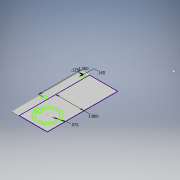
# Autodesk Inventor part: Power Button Plate
Saved by Autodesk Inventor 2019 (Build 230136000, 136)
## iProperties
Created: 2019-02-07
Part Number: Power Button Plate
Material: Generic
Document SubType Name: Modeling
Designer: mrhftc
Density: 1 g/cm^3
Appearance: Default
Author: mrhftc
Autodesk Inventor part; units mm, degrees
ref_plane "YZ Plane" through (0, 0, 0) normal (1, 0, 0) x (0, 1, 0)
ref_plane "XZ Plane" through (0, 0, 0) normal (0, 1, 0) x (-1, 0, 0)
ref_plane "XY Plane" through (0, 0, 0) normal (0, 0, 1) x (1, 0, 0)
sketch "Sketch1" plane through (0, 0, 0) normal (0, 1, 0) x (-1, 0, 0)
  line L0 (9.9313, 40.7784) -> (41.6813, 40.7784)
  line L1 (41.6813, 40.7784) -> (41.6813, 104.2784)
  line L2 (41.6813, 104.2784) -> (9.9313, 104.2784)
  line L3 (9.9313, 104.2784) -> (9.9313, 40.7784)
  point P0 (0, 0)
  dimension "d0" = 63.5
  dimension "d1" = 31.75
  constraints: 8 end point, 2 parallel, 1 horizontal, 1 perpendicular
  measures "d0" distance between parallel lines of L0 L2
  measures "d1" distance between parallel lines of L3 L1
extrude "Extrusion1" add sketch "Sketch1" along normal blind 0.3175
sketch "Sketch2" plane through (0, 0.3175, 0) normal (0, 1, 0) x (1, 0, 0)
  line L0 (-9.9313, -40.7784) -> (-41.6813, -40.7784) construction
  line L1 (-41.6813, -40.7784) -> (-41.6813, -104.2784) construction
  line L2 (-41.6813, -104.2784) -> (-9.9313, -104.2784) construction
  line L3 (-9.9313, -104.2784) -> (-9.9313, -40.7784) construction
  line L4 (-9.9313, -104.2784) -> (-35.3313, -104.2784)
  line L5 (-35.3313, -104.2784) -> (-35.3313, -40.7784)
  line L6 (-35.3313, -40.7784) -> (-9.9313, -40.7784)
  line L7 (-9.9313, -40.7784) -> (-9.9313, -104.2784)
  circle A0 centre (-38.5063, -44.3234) radius 2.1
  circle A1 centre (-38.5063, -78.8784) radius 2.1
  circle A2 centre (-22.6313, -91.3891) radius 9.9597
  circle A3 centre (-22.6313, -91.3891) radius 8.0547
  line L8 (-33.8243, -93.0121) -> (-28.1867, -93.0121)
  line L9 (-28.1867, -93.0121) -> (-28.1867, -90.0224)
  line L10 (-28.1867, -90.0224) -> (-33.8243, -90.0224)
  line L11 (-33.8243, -90.0224) -> (-33.8243, -93.0121)
  point P0 (0, 0)
  dimension "d4" = 25.4
  dimension "d5" = 3.175
  dimension "d6" = 4.2
  dimension "d7" = 38.1
  dimension "d8" = 1.905
  constraints: 16 end point, 4 centre point, 4 parallel, 2 horizontal, 2 perpendicular, 1 coincident, 1 point on line
  measures "d4" distance between parallel lines of L3 L5
  measures "d5" distance from line of L1 A0.centre
  measures "d6" diameter of A0
  measures "d7" distance from line of L0 A1.centre
  measures "d8" radial gap between concentric circles of A2 A3
body "Solid1"
